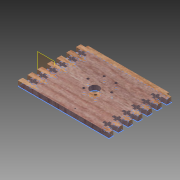
# Autodesk Inventor part: stepperMotorMountPlate01resized01
Saved by Autodesk Inventor 2013 (Build 170138000, 138)
## iProperties
Created: 2013-02-23
Part Number: stepperMotorMountPlate01resized01
Material: Wood (Birch)
Document SubType Name: Modeling
Designer: Nano
Density: 0.55 g/cm^3
Mass: 20.9125 g
Surface Area: 257.148 cm^2
Volume: 38.0226 cm^3
Author: Nano
Autodesk Inventor part; units mm, degrees
ref_plane "YZ Plane" through (0, 0, 0) normal (1, 0, 0) x (0, 1, 0)
ref_plane "XZ Plane" through (0, 0, 0) normal (0, 1, 0) x (-1, 0, 0)
ref_plane "XY Plane" through (0, 0, 0) normal (0, 0, 1) x (1, 0, 0)
sketch "Sketch1" plane through (0, 0, 0) normal (0, 1, 0) x (-1, 0, 0)
  line L0 (64.0604, 50.8) -> (-62.9396, 50.8)
  line L1 (-62.9396, 50.8) -> (-62.9396, -50.8)
  line L2 (-62.9396, -50.8) -> (64.0604, -50.8)
  line L3 (64.0604, -50.8) -> (64.0604, 50.8)
  line L4 (0, 0) -> (101.6, 0) construction
  line L5 (0, 50.8) -> (0, -50.8) construction
  line L6 (-58.3406, 0) -> (58.3406, 0) construction
  circle A0 centre (0, 0) radius 6
  circle A1 centre (-15.5097, -7.0044) radius 1.5875
  circle A2 centre (15.5097, -7.0044) radius 1.5875
  circle A3 centre (7.7597, 6.419) radius 1.5875
  circle A4 centre (7.7597, -20.4278) radius 1.5875
  circle A5 centre (-7.75, 6.4234) radius 1.5875
  circle A6 centre (-7.75, -20.4234) radius 1.5875
  arc A7 (1.7433, -2.4415) -> (-1.8557, -2.3572) centre (0, 0) ccw
  point P0 (0, 0)
  point P1 (0, 0)
  dimension "d1" = 127
  dimension "d2" = 101.6
  dimension "d31" = 12
  dimension "d32" = 0
  dimension "d33" = 3.175
  dimension "d34" = 17.018
  dimension "d35" = 3.175
  dimension "d36" = 17.018
  dimension "d37" = 3.175
  dimension "d38" = 3.175
  dimension "d39" = 10.0706
  dimension "d40" = 21.8519
  dimension "d41" = 15.5
  dimension "d42" = 15.5
  constraints: 14 end point, 8 centre point, 2 coincident, 2 horizontal, 2 parallel, 2 point on circle, 1 midpoint, 1 perpendicular, 1 vertical
  measures "d1" distance of L0.start L0.end
  measures "d2" distance of L1.end L0.end
  measures "d31" diameter of A0
  measures "d32" distance of point (0, 0) A0.centre
  measures "d33" diameter of A1
  measures "d34" distance of point (0, 0) A1.centre
  measures "d35" diameter of A2
  measures "d36" distance of point (0, 0) A2.centre
  measures "d37" diameter of A3
  measures "d38" diameter of A4
  measures "d39" distance of A3.centre point (0, 0)
  measures "d40" distance of A4.centre point (0, 0)
  measures "d41" distance of A4.centre A2.centre
  measures "d42" distance of A2.centre A3.centre
extrude "Extrusion1" add sketch "Sketch1" along normal blind 6.35
ref_plane "Work Plane1" through (-64.0604, 0, 0) normal (0, 0, 1) x (1, 0, 0)
sketch "Sketch4" plane through (0, 0, 0) normal (0, -1, 0) x (1, 0, 0)
  line L0 (-59.5312, 50.8) -> (59.5312, 50.8)
  line L1 (59.5312, 50.8) -> (59.5312, 41.0053)
  line L2 (59.5312, 41.0053) -> (-59.5312, 41.0053)
  line L3 (-59.5312, 41.0053) -> (-59.5312, 50.8)
  constraints: 8 end point, 2 parallel, 1 horizontal, 1 perpendicular
extrude "Extrusion4" cut sketch "Sketch4" against normal through all
sketch "Sketch5" plane through (0, 6.35, 0) normal (0, 1, 0) x (1, 0, 0)
  line L0 (-53.1588, 44.45) -> (53.205, 44.45)
  line L1 (-53.1588, 44.45) -> (-53.1588, 41.275)
  line L2 (-53.1588, 41.275) -> (-59.5131, 41.275)
  line L3 (-59.5131, 34.925) -> (-59.5131, 41.275)
  line L4 (-59.5131, 34.925) -> (-53.1588, 34.925)
  line L5 (-53.1588, 34.925) -> (-53.1588, 33.3375)
  line L6 (-53.1588, 33.3375) -> (-50.3806, 33.3375)
  line L7 (-50.3806, 33.3375) -> (-50.3806, 35.7188)
  line L8 (-50.3806, 35.7188) -> (-47.2056, 35.7188)
  line L9 (-47.2056, 35.7188) -> (-47.2056, 33.3375)
  line L10 (-47.2056, 33.3375) -> (-43.1262, 33.3375)
  line L11 (-43.1262, 33.3375) -> (-43.1262, 30.1625)
  line L12 (-43.1262, 30.1625) -> (-47.2056, 30.1625)
  line L13 (-47.2056, 30.1625) -> (-47.2056, 27.7813)
  line L14 (-47.2056, 27.7813) -> (-50.3806, 27.7813)
  line L15 (-50.3806, 27.7813) -> (-50.3806, 30.1625)
  line L16 (-50.3806, 30.1625) -> (-53.1588, 30.1625)
  line L17 (-53.1588, 30.1625) -> (-53.1588, 28.575)
  line L18 (-53.1588, 28.575) -> (-59.5131, 28.575)
  line L19 (-59.5131, 22.225) -> (-59.5131, 28.575)
  line L20 (-59.5131, 22.225) -> (-53.1588, 22.225)
  line L21 (-53.1588, 22.225) -> (-53.1588, 20.6375)
  line L22 (-53.1588, 20.6375) -> (-50.3806, 20.6375)
  line L23 (-50.3806, 20.6375) -> (-50.3806, 23.0188)
  line L24 (-50.3806, 23.0188) -> (-47.2056, 23.0188)
  line L25 (-47.2056, 23.0188) -> (-47.2056, 20.6375)
  line L26 (-47.2056, 20.6375) -> (-43.1262, 20.6375)
  line L27 (-43.1262, 20.6375) -> (-43.1262, 17.4625)
  line L28 (-43.1262, 17.4625) -> (-47.2238, 17.4625)
  line L29 (-47.2238, 17.4625) -> (-47.2238, 15.0813)
  line L30 (-47.2238, 15.0813) -> (-50.3988, 15.0813)
  line L31 (-50.3988, 15.0813) -> (-50.3988, 17.4625)
  line L32 (-50.3988, 17.4625) -> (-53.1769, 17.4625)
  line L33 (-53.1769, 17.4625) -> (-53.1769, 15.875)
  line L34 (-53.1769, 15.875) -> (-59.5313, 15.875)
  line L35 (-59.5313, 9.525) -> (-59.5313, 15.875)
  line L36 (-59.5313, 9.525) -> (-53.1588, 9.525)
  line L37 (-53.1588, 9.525) -> (-53.1588, 7.9375)
  line L38 (-53.1588, 7.9375) -> (-50.3806, 7.9375)
  line L39 (-50.3806, 7.9375) -> (-50.3806, 10.3188)
  line L40 (-50.3806, 10.3188) -> (-47.2056, 10.3188)
  line L41 (-47.2056, 10.3188) -> (-47.2056, 7.9375)
  line L42 (-47.2056, 7.9375) -> (-43.1262, 7.9375)
  line L43 (-43.1262, 7.9375) -> (-43.1262, 4.7625)
  line L44 (-43.1262, 4.7625) -> (-47.2056, 4.7625)
  line L45 (-47.2056, 4.7625) -> (-47.2056, 2.3813)
  line L46 (-47.2056, 2.3813) -> (-50.3806, 2.3813)
  line L47 (-50.3806, 2.3813) -> (-50.3806, 4.7625)
  line L48 (-50.3806, 4.7625) -> (-53.1588, 4.7625)
  line L49 (-53.1588, 4.7625) -> (-53.1588, 3.175)
  line L50 (-53.1588, 3.175) -> (-59.5131, 3.175)
  line L51 (-59.5131, -3.175) -> (-59.5131, 3.175)
  line L52 (-59.5131, -3.175) -> (-53.1588, -3.175)
  line L53 (-53.1588, -3.175) -> (-53.1588, -4.7625)
  line L54 (-53.1588, -4.7625) -> (-50.3806, -4.7625)
  line L55 (-50.3806, -4.7625) -> (-50.3806, -2.3812)
  line L56 (-50.3806, -2.3812) -> (-47.2056, -2.3812)
  line L57 (-47.2056, -2.3812) -> (-47.2056, -4.7625)
  line L58 (-47.2056, -4.7625) -> (-43.1262, -4.7625)
  line L59 (-43.1262, -4.7625) -> (-43.1262, -7.9375)
  line L60 (-43.1262, -7.9375) -> (-47.2056, -7.9375)
  line L61 (-47.2056, -7.9375) -> (-47.2056, -10.3187)
  line L62 (-47.2056, -10.3187) -> (-50.3806, -10.3187)
  line L63 (-50.3806, -10.3187) -> (-50.3806, -7.9375)
  line L64 (-50.3806, -7.9375) -> (-53.1588, -7.9375)
  line L65 (-53.1588, -7.9375) -> (-53.1588, -9.525)
  line L66 (-53.1588, -9.525) -> (-59.5131, -9.525)
  line L67 (-59.5131, -15.875) -> (-59.5131, -9.525)
  line L68 (-59.5131, -15.875) -> (-53.1588, -15.875)
  line L69 (-53.1588, -15.875) -> (-53.1588, -17.4625)
  line L70 (-53.1588, -17.4625) -> (-50.3806, -17.4625)
  line L71 (-50.3806, -17.4625) -> (-50.3806, -15.0812)
  line L72 (-50.3806, -15.0812) -> (-47.2056, -15.0812)
  line L73 (-47.2056, -15.0812) -> (-47.2056, -17.4625)
  line L74 (-47.2056, -17.4625) -> (-43.1262, -17.4625)
  line L75 (-43.1262, -17.4625) -> (-43.1262, -20.6375)
  line L76 (-43.1262, -20.6375) -> (-47.2056, -20.6375)
  line L77 (-47.2056, -20.6375) -> (-47.2056, -23.0187)
  line L78 (-47.2056, -23.0187) -> (-50.3806, -23.0187)
  line L79 (-50.3806, -23.0187) -> (-50.3806, -20.6375)
  line L80 (-50.3806, -20.6375) -> (-53.1588, -20.6375)
  line L81 (-53.1588, -20.6375) -> (-53.1588, -22.225)
  line L82 (-53.1588, -22.225) -> (-59.5131, -22.225)
  line L83 (-59.5131, -28.575) -> (-59.5131, -22.225)
  line L84 (-59.5131, -28.575) -> (-53.1588, -28.575)
  line L85 (-53.1588, -28.575) -> (-53.1588, -30.1625)
  line L86 (-53.1588, -30.1625) -> (-50.3806, -30.1625)
  line L87 (-50.3806, -30.1625) -> (-50.3806, -27.7812)
  line L88 (-50.3806, -27.7812) -> (-47.2056, -27.7812)
  line L89 (-47.2056, -27.7812) -> (-47.2056, -30.1625)
  line L90 (-47.2056, -30.1625) -> (-43.1262, -30.1625)
  line L91 (-43.1262, -30.1625) -> (-43.1262, -33.3375)
  line L92 (-43.1262, -33.3375) -> (-47.2056, -33.3375)
  line L93 (-47.2056, -33.3375) -> (-47.2056, -35.7187)
  line L94 (-47.2056, -35.7187) -> (-50.3806, -35.7187)
  line L95 (-50.3806, -35.7187) -> (-50.3806, -33.3375)
  line L96 (-50.3806, -33.3375) -> (-53.1588, -33.3375)
  line L97 (-53.1588, -33.3375) -> (-53.1588, -34.925)
  line L98 (-53.1588, -34.925) -> (-59.5131, -34.925)
  line L99 (-59.5131, -41.275) -> (-59.5131, -34.925)
  line L100 (-59.5131, -41.275) -> (-53.1588, -41.275)
  line L101 (-53.1588, -41.275) -> (-53.1588, -44.45)
  line L102 (53.205, -44.45) -> (-53.1588, -44.45)
  line L103 (59.5312, -270.0967) -> (59.5312, 14.8899) projected
  line L104 (-59.5313, 14.8899) -> (-59.5313, 87.2619) construction
  line L105 (59.5312, 14.8899) -> (59.5312, 87.2619) construction
  line L106 (0, 88.6989) -> (0, -326.401) construction
  line L107 (53.205, 44.45) -> (53.205, 41.275)
  line L108 (53.205, 41.275) -> (59.5131, 41.275)
  line L109 (59.5131, 34.925) -> (59.5131, 41.275)
  line L110 (59.5131, 34.925) -> (53.205, 34.925)
  line L111 (53.205, 34.925) -> (53.205, 33.3375)
  line L112 (53.205, 33.3375) -> (50.4269, 33.3375)
  line L113 (50.4269, 33.3375) -> (50.4269, 35.7188)
  line L114 (50.4269, 35.7188) -> (47.2519, 35.7188)
  line L115 (47.2519, 35.7188) -> (47.2519, 33.3375)
  line L116 (47.2519, 33.3375) -> (43.1724, 33.3375)
  line L117 (43.1724, 33.3375) -> (43.1724, 30.1625)
  line L118 (43.1724, 30.1625) -> (47.2519, 30.1625)
  line L119 (47.2519, 30.1625) -> (47.2519, 27.7813)
  line L120 (47.2519, 27.7813) -> (50.4269, 27.7813)
  line L121 (50.4269, 27.7813) -> (50.4269, 30.1625)
  line L122 (50.4269, 30.1625) -> (53.205, 30.1625)
  line L123 (53.205, 30.1625) -> (53.205, 28.575)
  line L124 (53.205, 28.575) -> (59.5131, 28.575)
  line L125 (59.5131, 22.225) -> (59.5131, 28.575)
  line L126 (59.5131, 22.225) -> (53.205, 22.225)
  line L127 (53.205, 22.225) -> (53.205, 20.6375)
  line L128 (53.205, 20.6375) -> (50.4269, 20.6375)
  line L129 (50.4269, 20.6375) -> (50.4269, 23.0188)
  line L130 (50.4269, 23.0188) -> (47.2519, 23.0188)
  line L131 (47.2519, 23.0188) -> (47.2519, 20.6375)
  line L132 (47.2519, 20.6375) -> (43.1724, 20.6375)
  line L133 (43.1724, 20.6375) -> (43.1724, 17.4625)
  line L134 (43.1724, 17.4625) -> (47.27, 17.4625)
  line L135 (47.27, 17.4625) -> (47.27, 15.0813)
  line L136 (47.27, 15.0813) -> (50.445, 15.0813)
  line L137 (50.445, 15.0813) -> (50.445, 17.4625)
  line L138 (50.445, 17.4625) -> (53.2232, 17.4625)
  line L139 (53.2232, 17.4625) -> (53.2232, 15.875)
  line L140 (53.2232, 15.875) -> (59.5312, 15.875)
  line L141 (59.5312, 9.525) -> (59.5312, 15.875)
  line L142 (59.5312, 9.525) -> (53.205, 9.525)
  line L143 (53.205, 9.525) -> (53.205, 7.9375)
  line L144 (53.205, 7.9375) -> (50.4269, 7.9375)
  line L145 (50.4269, 7.9375) -> (50.4269, 10.3188)
  line L146 (50.4269, 10.3188) -> (47.2519, 10.3188)
  line L147 (47.2519, 10.3188) -> (47.2519, 7.9375)
  line L148 (47.2519, 7.9375) -> (43.1724, 7.9375)
  line L149 (43.1724, 7.9375) -> (43.1724, 4.7625)
  line L150 (43.1724, 4.7625) -> (47.2519, 4.7625)
  line L151 (47.2519, 4.7625) -> (47.2519, 2.3813)
  line L152 (47.2519, 2.3813) -> (50.4269, 2.3813)
  line L153 (50.4269, 2.3813) -> (50.4269, 4.7625)
  line L154 (50.4269, 4.7625) -> (53.205, 4.7625)
  line L155 (53.205, 4.7625) -> (53.205, 3.175)
  line L156 (53.205, 3.175) -> (59.5131, 3.175)
  line L157 (59.5131, -3.175) -> (59.5131, 3.175)
  line L158 (59.5131, -3.175) -> (53.205, -3.175)
  line L159 (53.205, -3.175) -> (53.205, -4.7625)
  line L160 (53.205, -4.7625) -> (50.4269, -4.7625)
  line L161 (50.4269, -4.7625) -> (50.4269, -2.3812)
  line L162 (50.4269, -2.3812) -> (47.2519, -2.3812)
  line L163 (47.2519, -2.3812) -> (47.2519, -4.7625)
  line L164 (47.2519, -4.7625) -> (43.1724, -4.7625)
  line L165 (43.1724, -4.7625) -> (43.1724, -7.9375)
  line L166 (43.1724, -7.9375) -> (47.2519, -7.9375)
  line L167 (47.2519, -7.9375) -> (47.2519, -10.3187)
  line L168 (47.2519, -10.3187) -> (50.4269, -10.3187)
  line L169 (50.4269, -10.3187) -> (50.4269, -7.9375)
  line L170 (50.4269, -7.9375) -> (53.205, -7.9375)
  line L171 (53.205, -7.9375) -> (53.205, -9.525)
  line L172 (53.205, -9.525) -> (59.5131, -9.525)
  line L173 (59.5131, -15.875) -> (59.5131, -9.525)
  line L174 (59.5131, -15.875) -> (53.205, -15.875)
  line L175 (53.205, -15.875) -> (53.205, -17.4625)
  line L176 (53.205, -17.4625) -> (50.4269, -17.4625)
  line L177 (50.4269, -17.4625) -> (50.4269, -15.0812)
  line L178 (50.4269, -15.0812) -> (47.2519, -15.0812)
  line L179 (47.2519, -15.0812) -> (47.2519, -17.4625)
  line L180 (47.2519, -17.4625) -> (43.1724, -17.4625)
  line L181 (43.1724, -17.4625) -> (43.1724, -20.6375)
  line L182 (43.1724, -20.6375) -> (47.2519, -20.6375)
  line L183 (47.2519, -20.6375) -> (47.2519, -23.0187)
  line L184 (47.2519, -23.0187) -> (50.4269, -23.0187)
  line L185 (50.4269, -23.0187) -> (50.4269, -20.6375)
  line L186 (50.4269, -20.6375) -> (53.205, -20.6375)
  line L187 (53.205, -20.6375) -> (53.205, -22.225)
  line L188 (53.205, -22.225) -> (59.5131, -22.225)
  line L189 (59.5131, -28.575) -> (59.5131, -22.225)
  line L190 (59.5131, -28.575) -> (53.205, -28.575)
  line L191 (53.205, -28.575) -> (53.205, -30.1625)
  line L192 (53.205, -30.1625) -> (50.4269, -30.1625)
  line L193 (50.4269, -30.1625) -> (50.4269, -27.7812)
  line L194 (50.4269, -27.7812) -> (47.2519, -27.7812)
  line L195 (47.2519, -27.7812) -> (47.2519, -30.1625)
  line L196 (47.2519, -30.1625) -> (43.1724, -30.1625)
  line L197 (43.1724, -30.1625) -> (43.1724, -33.3375)
  line L198 (43.1724, -33.3375) -> (47.2519, -33.3375)
  line L199 (47.2519, -33.3375) -> (47.2519, -35.7187)
  line L200 (47.2519, -35.7187) -> (50.4269, -35.7187)
  line L201 (50.4269, -35.7187) -> (50.4269, -33.3375)
  line L202 (50.4269, -33.3375) -> (53.205, -33.3375)
  line L203 (53.205, -33.3375) -> (53.205, -34.925)
  line L204 (53.205, -34.925) -> (59.5131, -34.925)
  line L205 (59.5131, -41.275) -> (59.5131, -34.925)
  line L206 (59.5131, -41.275) -> (53.205, -41.275)
  line L207 (53.205, -41.275) -> (53.205, -44.45)
  line L208 (-59.5312, -41.0053) -> (59.5312, -41.0053) projected
  line L209 (-53.1813, 87.2619) -> (-53.1813, 14.8899) projected
  point P0 (-58.3406, -41.0053)
  point P1 (58.3406, -41.0053)
  constraints: 410 end point, 1 point on line, 1 vertical, 2 other
extrude "Extrusion7" cut sketch "Sketch5" against normal blind 25.4 contours L0 L107 L108 L109 L110 L111 L112 L113 L114 L115 L116 L117 L118 L119 L120 L121 L122 L123 L124 L125 L126 L127 L128 L129 L130 L131 L132 L133 L134 L135 L136 L137 L138 L139 L140 L141 L103 L142 L143 L144 L145 L146 L147 L148 L149 L150 L151 L152 L153 L154 L155 L156 L157 L158 L159 L160 L161 L162 L163 L164 L165 L166 L167 L168 L169 L170 L171 L172 L173 L174 L175 L176 L177 L178 L179 L180 L181 L182 L183 L184 L185 L186 L187 L188 L189 L190 L191 L192 L193 L194 L195 L196 L197 L198 L199 L200 L201 L202 L203 L204 L205 L208 L99 L98 L97 L96 L95 L94 L93 L92 L91 L90 L89 L88 L87 L86 L85 L84 L83 L82 L81 L80 L79 L78 L77 L76 L75 L74 L73 L72 L71 L70 L69 L68 L67 L66 L65 L64 L63 L62 L61 L60 L59 L58 L57 L56 L55 L54 L53 L52 L51 L50 L49 L48 L47 L46 L45 L44 L43 L42 L41 L40 L39 L38 L37 L36 L35 L34 L33 L32 L31 L30 L29 L28 L27 L26 L25 L24 L23 L22 L21 L20 L209 L18 L17 L16 L15 L14 L13 L12 L11 L10 L9 L8 L7 L6 L5 L4 L2 L1 | L209 L4 L3 L2 | L209 L20 L19 L18 | L205 L206 L207 L102 L101 L100 L99 L208 keep common part
equation "\"d42\" = d41"
body "Solid1"
